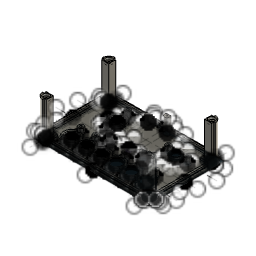
Cover_top v19 final (Autodesk Fusion 360 design; units mm, degrees)
Autodesk Fusion 360 part; units mm, degrees
(part 1 of 2)
sketch "Skizze1" plane through (0, 0, 0) normal (0, 0, 1) x (1, 0, 0)
  line L0 (85, -55) -> (-85, -55)
  line L1 (-85, -55) -> (-85, 55)
  line L2 (-85, 55) -> (85, 55)
  line L3 (85, 55) -> (85, -55)
  line L4 (85, -55) -> (-85, 55) construction
  line L5 (-85, -55) -> (85, 55) construction
  circle A0 centre (-75, 45) radius 10
  circle A1 centre (-75, -45) radius 10
  circle A2 centre (75, 45) radius 10
  line L6 (83.8, -53.8) -> (-83.8, -53.8)
  line L7 (-83.8, -53.8) -> (-83.8, 53.8)
  line L8 (-83.8, 53.8) -> (83.8, 53.8)
  line L9 (83.8, 53.8) -> (83.8, -53.8)
  line L10 (83.8, -53.8) -> (-83.8, 53.8) construction
  line L11 (-83.8, -53.8) -> (83.8, 53.8) construction
  line L12 (-70.8, 53.8) -> (-83.8, 53.8)
  line L13 (-83.8, 53.8) -> (-83.8, 40.8)
  line L14 (-83.8, 40.8) -> (-70.8, 40.8)
  line L15 (-70.8, 40.8) -> (-70.8, 53.8)
  line L16 (-83.8, 36) -> (-83.8, 45.2283)
  line L17 (-83.8, -40.8) -> (-70.8, -40.8)
  line L18 (-70.8, -40.8) -> (-70.8, -53.8)
  line L19 (-70.8, -53.8) -> (-83.8, -53.8)
  line L20 (-83.8, -53.8) -> (-83.8, -40.8)
  line L21 (83.8, -40.8) -> (70.8, -40.8)
  line L22 (70.8, -40.8) -> (70.8, -53.8)
  line L23 (70.8, -53.8) -> (83.8, -53.8)
  line L24 (83.8, -53.8) -> (83.8, -40.8)
  line L25 (70.8, 53.8) -> (83.8, 53.8)
  line L26 (83.8, 53.8) -> (83.8, 40.8)
  line L27 (83.8, 40.8) -> (70.8, 40.8)
  line L28 (70.8, 40.8) -> (70.8, 53.8)
  line L29 (-107.8935, 0) -> (101.4161, 0) construction
  line L30 (-81.6, -44) -> (-83.8, -44)
  line L31 (-83.8, -44) -> (-83.8, 44)
  line L32 (-83.8, 44) -> (-81.6, 44)
  line L33 (-81.6, 44) -> (-81.6, -44)
  line L34 (-81.6, -44) -> (-83.8, 44) construction
  line L35 (-83.8, -44) -> (-81.6, 44) construction
  line L36 (74, 51.6) -> (-74, 51.6)
  line L37 (-74, 51.6) -> (-74, 53.8)
  line L38 (-74, 53.8) -> (74, 53.8)
  line L39 (74, 53.8) -> (74, 51.6)
  line L40 (74, 51.6) -> (-74, 53.8) construction
  line L41 (-74, 51.6) -> (74, 53.8) construction
  line L42 (0, 66.6511) -> (0, -64.6622) construction
  line L43 (-89.5499, 46.3) -> (95, 46.3) construction
  line L44 (-93.2916, -46.3) -> (96.8462, -46.3) construction
  line L45 (-76.3, 67.4333) -> (-76.3, -70) construction
  line L46 (76.3, 67.4333) -> (76.3, -68.5532) construction
  circle A3 centre (76.3, -46.3) radius 4.5
  circle A4 centre (76.3, -46.3) radius 3
  circle A5 centre (76.3, 46.3) radius 4.5
  circle A6 centre (76.3, 46.3) radius 3
  circle A7 centre (-76.3, 46.3) radius 4.5
  circle A8 centre (-76.3, 46.3) radius 3
  circle A9 centre (-76.3, -46.3) radius 4.5
  circle A10 centre (-76.3, -46.3) radius 3
  line L47 (83.8, -44) -> (81.6, -44)
  line L48 (81.6, -44) -> (81.6, 44)
  line L49 (81.6, 44) -> (83.8, 44)
  line L50 (83.8, 44) -> (83.8, -44)
  line L51 (83.8, -44) -> (81.6, 44) construction
  line L52 (81.6, -44) -> (83.8, 44) construction
  line L53 (74, -53.8) -> (-74, -53.8)
  line L54 (-74, -53.8) -> (-74, -51.6)
  line L55 (-74, -51.6) -> (74, -51.6)
  line L56 (74, -51.6) -> (74, -53.8)
  line L57 (74, -53.8) -> (-74, -51.6) construction
  line L58 (-74, -53.8) -> (74, -51.6) construction
  line L59 (-95.9199, -30) -> (100, -30) construction
  line L60 (-91.3971, -16.03) -> (91.4123, -16.03) construction
  line L61 (-89.9566, -43.97) -> (89.6836, -43.97) construction
  line L62 (-11, 2.8713) -> (-11, -37.609) construction
  line L63 (-33, 11.0826) -> (-33, -38.4733) construction
  line L64 (-55, 10.5064) -> (-55, -36.1684) construction
  line L65 (11, 3.8797) -> (11, -36.4565) construction
  line L66 (33, 5.4644) -> (33, -35) construction
  line L67 (55, 5.8965) -> (55, -33.5753) construction
  circle A11 centre (-55, -30) radius 12
  circle A12 centre (-33, -30) radius 12
  circle A13 centre (-11, -30) radius 12
  circle A14 centre (11, -30) radius 12
  circle A15 centre (33, -30) radius 12
  circle A16 centre (55, -30) radius 12
  circle A17 centre (55, -16.03) radius 4
  circle A18 centre (33, -16.03) radius 4
  circle A19 centre (11, -16.03) radius 4
  circle A20 centre (-11, -16.03) radius 4
  circle A21 centre (-33, -16.03) radius 4
  circle A22 centre (-55, -16.03) radius 4
  circle A23 centre (-55, -43.97) radius 4
  circle A24 centre (-33, -43.97) radius 4
  circle A25 centre (-11, -43.97) radius 4
  circle A26 centre (11, -43.97) radius 4
  circle A27 centre (33, -43.97) radius 4
  circle A28 centre (55, -43.97) radius 4
  circle A29 centre (55, -30) radius 9.1
  circle A30 centre (55, -30) radius 8.1
  circle A31 centre (33, -30) radius 9.1
  circle A32 centre (33, -30) radius 8.1
  circle A33 centre (11, -30) radius 9.1
  circle A34 centre (11, -30) radius 8.1
  circle A35 centre (-11, -30) radius 9.1
  circle A36 centre (-11, -30) radius 8.1
  circle A37 centre (-33, -30) radius 9.1
  circle A38 centre (-33, -30) radius 8.1
  circle A39 centre (-55, -30) radius 9.1
  circle A40 centre (-55, -30) radius 8.1
  line L68 (-67.8, 37.8) -> (-67.8, 48.6)
  line L69 (-67.8, 48.6) -> (67.8, 48.6)
  line L70 (67.8, 48.6) -> (67.8, 37.8)
  line L71 (67.8, 37.8) -> (78.6, 37.8)
  line L72 (78.6, 37.8) -> (78.6, -37.8)
  line L73 (78.6, -37.8) -> (67.8, -37.8)
  line L74 (67.8, -37.8) -> (67.8, -48.6)
  line L75 (67.8, -48.6) -> (-67.8, -48.6)
  line L76 (-67.8, -48.6) -> (-67.8, -38.0603)
  line L77 (-67.8, -38.0603) -> (-78.6, -38.0603)
  line L78 (-78.6, -38.0603) -> (-78.6, 37.8)
  line L79 (-78.6, 37.8) -> (-67.8, 37.8)
  line L80 (-100.7551, 25) -> (105, 25) construction
  line L81 (44.54, 42.8921) -> (44.54, 3.8544) construction
  line L82 (-42, 44.1013) -> (-42, 5.0635) construction
  circle A41 centre (-42, 25) radius 9.1
  circle A42 centre (-42, 25) radius 8.1
  circle A43 centre (-42, 25) radius 12
  line L83 (-48.7348, 40.24) -> (-29.0042, 40.24) construction
  line L84 (-50, 9.76) -> (-24.2465, 9.76) construction
  circle A44 centre (-42, 40.24) radius 4
  circle A45 centre (-42, 9.76) radius 4
  circle A46 centre (44.54, 25) radius 6.25
  circle A47 centre (44.54, 25) radius 7.5
  line L85 (61.54, 32) -> (61.54, 15) construction
  line L86 (33.54, 36) -> (33.54, 15.2872) construction
  circle A48 centre (33.54, 25) radius 4
  circle A49 centre (61.54, 25) radius 4
  line L87 (-55.79, 35.0443) -> (-55.79, 15.0443) construction
  circle A50 centre (-55.79, 25) radius 3.25
  circle A51 centre (-55.79, 25) radius 1.75
  line L88 (-22.9425, -17) -> (36.8868, -17) construction
  line L89 (-26.9921, 49.1) -> (29.3101, 49.1) construction
  line L90 (-28, 65.5218) -> (-28, -4.3972) construction
  line L91 (-25.5, 61.3213) -> (-25.5, -3.5842) construction
  line L92 (-20.4, 60) -> (-20.4, -2) construction
  line L93 (7.5, 61) -> (7.5, 1) construction
  line L94 (22.7, 60.5796) -> (22.7, -4.8964) construction
  line L95 (3.5, 51.6) -> (11.5, 51.6)
  line L96 (11.5, 51.6) -> (11.5, 45.1) construction
  line L97 (11.5, 45.1) -> (3.5, 45.1) construction
  line L98 (3.5, 45.1) -> (3.5, 51.6) construction
  line L99 (-24.4, 51.6) -> (-16.4, 51.6)
  line L100 (-16.4, 51.6) -> (-16.4, 45.1) construction
  line L101 (-16.4, 45.1) -> (-24.4, 45.1) construction
  line L102 (-24.4, 45.1) -> (-24.4, 51.6) construction
  line L103 (-17.4, 51.6) -> (-17.4, 45.1)
  arc A52 (-24.4, 49.1) -> (-16.4, 49.1) centre (-20.4, 49.1) ccw
  arc A53 (-23.5225, 51.6) -> (-24.4, 49.1) centre (-20.4, 49.1) ccw
  arc A54 (-16.4, 49.1) -> (-17.2775, 51.6) centre (-20.4, 49.1) ccw
  arc A55 (3.5, 49.1) -> (10.6225, 51.6) centre (7.5, 49.1) ccw
  arc A56 (4.3775, 51.6) -> (3.5, 49.1) centre (7.5, 49.1) ccw
  line L104 (18, -1.7) -> (26.495, -1.7) construction
  line L105 (27, -3) -> (-31, -3) construction
  circle A57 centre (22.7, -1.7) radius 4
  circle A58 centre (-25.5, -3) radius 4
  line L106 (19.3593, 0.5) -> (26.0407, 0.5)
  line L107 (74.2, -53.6) -> (74.2, -51.4)
  line L108 (74.2, -51.4) -> (71, -51.4)
  line L109 (71, -51.4) -> (71, -41)
  line L110 (71, -41) -> (81.4, -41)
  line L111 (81.4, -41) -> (81.4, -44.2)
  line L112 (81.4, -44.2) -> (83.6, -44.2)
  line L113 (74, -54.6568) -> (74, -41.9102) construction
  line L114 (69.7927, -44) -> (87.5, -44) construction
  arc A59 (74, -53.8) -> (83.8, -44) centre (74, -44) ccw
  arc A60 (74.2, -53.6) -> (83.6, -44.2) centre (74, -44) ccw
  line L115 (72.8, -53.6) -> (76.6, -53.6) construction
  line L116 (83.6, -43.5) -> (83.6, -45.7322) construction
  circle A61 centre (75, -45) radius 10
  arc A62 (-83.6, -44.2) -> (-74.2, -53.6) centre (-74, -44) ccw
  line L117 (-74.2, -53.6) -> (-74.2, -51.4)
  line L118 (-74.2, -51.4) -> (-71, -51.4)
  line L119 (-71, -41) -> (-81.4, -41)
  line L120 (-81.4, -41) -> (-81.4, -44.2)
  line L121 (-81.4, -44.2) -> (-83.6, -44.2)
  line L122 (-71, -51.4) -> (-71, -41)
  arc A63 (-83.8, -44) -> (-74, -53.8) centre (-74, -44) ccw
  arc A64 (-74.2, 53.6) -> (-83.6, 44.2) centre (-74, 44) ccw
  line L123 (-74.2, 53.6) -> (-74.2, 51.4)
  line L124 (-74.2, 51.4) -> (-71, 51.4)
  line L125 (-71, 41) -> (-81.4, 41)
  line L126 (-81.4, 41) -> (-81.4, 44.2)
  line L127 (-81.4, 44.2) -> (-83.6, 44.2)
  line L128 (-71, 51.4) -> (-71, 41)
  arc A65 (-74, 53.8) -> (-83.8, 44) centre (-74, 44) ccw
  arc A66 (83.6, 44.2) -> (74.2, 53.6) centre (74, 44) ccw
  line L129 (74.2, 53.6) -> (74.2, 51.4)
  line L130 (74.2, 51.4) -> (71, 51.4)
  line L131 (71, 41) -> (81.4, 41)
  line L132 (81.4, 41) -> (81.4, 44.2)
  line L133 (81.4, 44.2) -> (83.6, 44.2)
  line L134 (71, 51.4) -> (71, 41)
  arc A67 (83.8, 44) -> (74, 53.8) centre (74, 44) ccw
  line L135 (-83.6, 44.2) -> (-83.8, 44.2)
  line L136 (-74.2, 53.6) -> (-74.2, 53.8)
  line L137 (74.2, 53.6) -> (74.2, 53.8)
  line L138 (83.6, 44.2) -> (83.8, 44.2)
  line L139 (83.6, -44.2) -> (83.8, -44.2)
  line L140 (74.2, -53.6) -> (74.2, -53.8)
  line L141 (-74.2, -53.6) -> (-74.2, -53.8)
  line L142 (-83.6, -44.2) -> (-83.8, -44.2)
  line L143 (-11.75, 70) -> (-11.75, 19) construction
  point P0 (-82.7, 0)
  point P1 (0, 52.7)
  point P2 (76.3, -46.3)
  point P3 (76.3, 46.3)
  point P4 (-76.3, 46.3)
  point P5 (-76.3, -46.3)
  point P6 (82.7, 0)
  point P7 (0, -52.7)
  point P8 (-55, -30)
  point P9 (-33, -30)
  point P10 (-11, -30)
  point P11 (11, -30)
  point P12 (33, -30)
  point P13 (55, -30)
  point P14 (-55, -16.03)
  point P15 (-33, -16.03)
  point P16 (-11, -16.03)
  point P17 (11, -16.03)
  point P18 (33, -16.03)
  point P19 (55, -16.03)
  point P20 (55, -43.97)
  point P21 (33, -43.97)
  point P22 (11, -43.97)
  point P23 (-11, -43.97)
  point P24 (-33, -43.97)
  point P25 (-55, -43.97)
  point P26 (-42, 25)
  point P27 (44.54, 25)
  point P28 (-42, 9.76)
  point P29 (-42, 40.24)
  point P30 (33.54, 25)
  point P31 (61.54, 25)
  point P32 (7.5, 49.1)
  point P33 (-20.4, 49.1)
  point P34 (-25.5, -3)
  point P35 (22.7, -1.7)
  point P36 (74.2, -44.2)
  point P37 (74, -44)
  point P38 (74.2, -53.6)
  point P39 (83.6, -44.2)
  dimension "d1" = 110
  dimension "d2" = 170
  dimension "d3" = 20
  dimension "d4" = 20
  dimension "d6" = 20
  dimension "d7" = 167.6
  dimension "d8" = 107.6
  dimension "d13" = 13
  dimension "d14" = 13
  dimension "d17" = 13
  dimension "d18" = 13
  dimension "d19" = 13
  dimension "d20" = 13
  dimension "d21" = 13
  dimension "d22" = 13
  dimension "d23" = 1.1
  dimension "d24" = 2.2
  dimension "d25" = 88
  dimension "d26" = 1.1
  dimension "d27" = 2.2
  dimension "d28" = 148
  dimension "d29" = 5.5
  dimension "d30" = 5.5
  dimension "d31" = 5.5
  dimension "d32" = 5.5
  dimension "d33" = 9
  dimension "d34" = 6
  dimension "d35" = 9
  dimension "d36" = 6
  dimension "d37" = 6
  dimension "d38" = 9
  dimension "d39" = 6
  dimension "d40" = 9
  dimension "d41" = 2.2
  dimension "d42" = 1.1
  dimension "d43" = 88
  dimension "d44" = 1.1
  dimension "d45" = 148
  dimension "d46" = 2.2
  dimension "d47" = 25
  dimension "d48" = 13.97
  dimension "d49" = 13.97
  dimension "d50" = 11
  dimension "d51" = 22
  dimension "d52" = 22
  dimension "d53" = 11
  dimension "d54" = 22
  dimension "d55" = 22
  dimension "d56" = 24
  dimension "d57" = 24
  dimension "d58" = 24
  dimension "d59" = 24
  dimension "d60" = 24
  dimension "d61" = 24
  dimension "d62" = 8
  dimension "d63" = 8
  dimension "d64" = 8
  dimension "d65" = 8
  dimension "d66" = 8
  dimension "d67" = 8
  dimension "d68" = 8
  dimension "d69" = 8
  dimension "d70" = 8
  dimension "d71" = 8
  dimension "d72" = 8
  dimension "d73" = 8
  dimension "d74" = 18.2
  dimension "d75" = 18.2
  dimension "d76" = 18.2
  dimension "d77" = 18.2
  dimension "d78" = 18.2
  dimension "d79" = 18.2
  dimension "d80" = 16.2
  dimension "d81" = 16.2
  dimension "d82" = 16.2
  dimension "d83" = 16.2
  dimension "d84" = 16.2
  dimension "d85" = 16.2
  dimension "d116" = 3
  dimension "d117" = 3
  dimension "d118" = 3
  dimension "d119" = 3
  dimension "d120" = 3
  dimension "d121" = 3
  dimension "d122" = 3
  dimension "d123" = 3
  dimension "d124" = 3
  dimension "d125" = 3
  dimension "d126" = 3
  dimension "d127" = 2.7397
  dimension "d130" = 30
  dimension "d131" = 42
  dimension "d132" = 44.54
  dimension "d133" = 18.2
  dimension "d134" = 16.2
  dimension "d135" = 24
  dimension "d136" = 15.24
  dimension "d137" = 15.24
  dimension "d138" = 8
  dimension "d139" = 8
  dimension "d140" = 12.5
  dimension "d141" = 15
  dimension "d142" = 17
  dimension "d143" = 11
  dimension "d144" = 8
  dimension "d145" = 8
  dimension "d214" = 6.5
  dimension "d215" = 3.5
  dimension "d220" = 135.6
  dimension "d221" = 5.5
  dimension "d222" = 5.5
  dimension "d223" = 7.5
  dimension "d224" = 3.2
  dimension "d225" = 13.79
  dimension "d227" = 66.1
  dimension "d228" = 68.6
  dimension "d229" = 2.5
  dimension "d230" = 28
  dimension "d231" = 2.5
  dimension "d232" = 5.1
  dimension "d233" = 27.9
  dimension "d234" = 15.2
  dimension "d235" = 48.2
  dimension "d236" = 4
  dimension "d237" = 4
  dimension "d238" = 4
  dimension "d240" = 4
  dimension "d241" = 4
  dimension "d242" = 4
  dimension "d243" = 3
  dimension "d244" = 50.8
  dimension "d245" = 1.3
  dimension "d246" = 8
  dimension "d247" = 8
  dimension "d248" = 2.2
  dimension "d256" = 49.1
  dimension "d279" = 76.3
  dimension "d282" = 46.3
  dimension "d306" = 0.2
  dimension "d307" = 0.2
  dimension "d308" = 0.2
  dimension "d309" = 0.2
  dimension "d312" = 0.2
  dimension "d313" = 0.2
  dimension "d314" = 0.2
  dimension "d315" = 0.2
  dimension "d316" = 20
  dimension "d333" = 3.2
  dimension "d334" = 14.2
  dimension "d335" = 14.2
  dimension "d336" = 92.6
  dimension "d337" = 11.36
  dimension "d338" = 16.25
  dimension "d339" = 62.25
  dimension "d340" = 32
  constraint horizontal L0
  constraint perpendicular L0 L1
  constraint parallel L0 L2
  constraint parallel L1 L3
  constraint coincident L4 origin
  constraint coincident L5 origin
  constraint tangent L2 A0
  constraint tangent L1 A0
  constraint tangent L1 A1
  constraint tangent L0 A1
  constraint tangent L2 A2
  constraint tangent L3 A2
  constraint horizontal L6
  constraint perpendicular L6 L7
  constraint parallel L6 L8
  constraint parallel L7 L9
  constraint coincident L10 origin
  constraint coincident L11 origin
  constraint horizontal L12
  constraint vertical L13
  constraint horizontal L14
  constraint vertical L15
  constraint coincident L7 L13.end
  constraint coincident L8 L12.start
  constraint vertical L16
  constraint coincident L7 L16.end
  constraint horizontal L17
  constraint vertical L18
  constraint horizontal L19
  constraint vertical L20
  constraint coincident L6 L18.end
  constraint coincident L7 L17.start
  constraint horizontal L21
  constraint vertical L22
  constraint horizontal L23
  constraint vertical L24
  constraint coincident L6 L22.end
  constraint coincident L9 L21.start
  constraint horizontal L25
  constraint vertical L26
  constraint horizontal L27
  constraint vertical L28
  constraint coincident L9 L26.end
  constraint coincident L8 L25.start
  constraint perpendicular L3 L29
  constraint coincident origin L29
  constraint horizontal L30
  constraint perpendicular L30 L31
  constraint parallel L30 L32
  constraint parallel L31 L33
  constraint coincident L34 P0
  constraint coincident L35 P0
  constraint coincident L29 P0
  constraint horizontal L36
  constraint perpendicular L36 L37
  constraint parallel L36 L38
  constraint parallel L37 L39
  constraint coincident L40 P1
  constraint coincident L41 P1
  constraint perpendicular L0 L42
  constraint coincident origin L42
  constraint coincident P1 L42
  constraint parallel L36 L43
  constraint perpendicular L1 L44
  constraint perpendicular L17 L45
  constraint perpendicular L0 L46
  constraint coincident L44 P2
  constraint coincident L46 P2
  constraint coincident P2 A3.centre
  constraint coincident L43 P3
  constraint coincident L46 P3
  constraint coincident P3 A5.centre
  constraint coincident L43 P4
  constraint coincident L45 P4
  constraint coincident P4 A7.centre
  constraint coincident L44 P5
  constraint coincident L45 P5
  constraint coincident P5 A9.centre
  constraint horizontal L47
  constraint perpendicular L47 L48
  constraint parallel L47 L49
  constraint parallel L48 L50
  constraint coincident L51 P6
  constraint coincident L52 P6
  constraint coincident L29 P6
  constraint horizontal L53
  constraint perpendicular L53 L54
  constraint parallel L53 L55
  constraint parallel L54 L56
  constraint coincident L57 P7
  constraint coincident L58 P7
  constraint coincident L42 P7
  constraint perpendicular L3 L59
  constraint perpendicular L3 L60
  constraint perpendicular L50 L61
  constraint perpendicular L44 L62
  constraint perpendicular L61 L63
  constraint perpendicular L61 L64
  constraint perpendicular L61 L65
  constraint perpendicular L60 L66
  constraint vertical L67
  constraint coincident L59 P8
  constraint coincident L64 P8
  constraint coincident L59 P9
  constraint coincident L63 P9
  constraint coincident L59 P10
  constraint coincident L62 P10
  constraint coincident L59 P11
  constraint coincident L65 P11
  constraint coincident L59 P12
  constraint coincident L66 P12
  constraint coincident L59 P13
  constraint coincident L67 P13
  constraint coincident L60 P14
  constraint coincident L64 P14
  constraint coincident L60 P15
  constraint coincident L63 P15
  constraint coincident L60 P16
  constraint coincident L62 P16
  constraint coincident L60 P17
  constraint coincident L65 P17
  constraint coincident L66 P18
  constraint coincident L60 P18
  constraint coincident L60 P19
  constraint coincident L67 P19
  constraint coincident L61 P20
  constraint coincident L67 P20
  constraint coincident L66 P21
  constraint coincident L61 P21
  constraint coincident L61 P22
  constraint coincident L65 P22
  constraint coincident L61 P23
  constraint coincident L62 P23
  constraint coincident L61 P24
  constraint coincident L63 P24
  constraint coincident L61 P25
  constraint coincident L64 P25
  constraint coincident P8 A11.centre
  constraint coincident P9 A12.centre
  constraint coincident P10 A13.centre
  constraint coincident P11 A14.centre
  constraint coincident P12 A15.centre
  constraint coincident P13 A16.centre
  constraint coincident P19 A17.centre
  constraint coincident P18 A18.centre
  constraint coincident P17 A19.centre
  constraint coincident P16 A20.centre
  constraint coincident P15 A21.centre
  constraint coincident P14 A22.centre
  constraint coincident P25 A23.centre
  constraint coincident P24 A24.centre
  constraint coincident P23 A25.centre
  constraint coincident P22 A26.centre
  constraint coincident P21 A27.centre
  constraint coincident P20 A28.centre
  constraint concentric A16 A29
  constraint concentric A15 A31
  constraint concentric A15 A32
  constraint concentric A14 A34
  constraint perpendicular L43 L68
  constraint perpendicular L28 L69
  constraint perpendicular L43 L70
  constraint perpendicular L46 L71
  constraint perpendicular L71 L72
  constraint perpendicular L46 L73
  constraint perpendicular L44 L74
  constraint perpendicular L74 L75
  constraint coincident A1 L76.end
  constraint perpendicular L75 L76
  constraint perpendicular L45 L77
  constraint perpendicular L77 L78
  constraint perpendicular L68 L79
  constraint perpendicular L3 L80
  constraint perpendicular L43 L81
  constraint coincident L80 P26
  constraint coincident L82 P26
  constraint coincident L80 P27
  constraint coincident L81 P27
  constraint coincident P26 A41.centre
  constraint perpendicular L45 L83
  constraint horizontal L84
  constraint coincident L82 P28
  constraint coincident L84 P28
  constraint coincident L82 P29
  constraint coincident L83 P29
  constraint coincident P29 A44.centre
  constraint coincident P28 A45.centre
  constraint coincident P27 A46.centre
  constraint perpendicular L80 L85
  constraint perpendicular L80 L86
  constraint coincident L80 P30
  constraint coincident L86 P30
  constraint coincident L80 P31
  constraint coincident L85 P31
  constraint coincident P30 A48.centre
  constraint coincident P31 A49.centre
  constraint perpendicular L80 L87
  constraint coincident L80 A50.centre
  constraint coincident L87 A50.centre
  constraint concentric A50 A51
  constraint perpendicular L66 L88
  constraint parallel L43 L89
  constraint perpendicular L2 L90
  constraint perpendicular L29 L91
  constraint perpendicular L29 L92
  constraint vertical L93
  constraint perpendicular L29 L94
  constraint horizontal L95
  constraint vertical L96
  constraint horizontal L97
  constraint vertical L98
  constraint coincident L36 L95.start
  constraint coincident L89 P32
  constraint coincident L93 P32
  constraint coincident L92 P33
  constraint coincident L89 P33
  constraint horizontal L99
  constraint vertical L100
  constraint horizontal L101
  constraint vertical L102
  constraint coincident L36 L99.start
  constraint coincident L36 L103.start
  constraint coincident L101 L103.end
  constraint perpendicular L101 L103
  constraint coincident L100 A52.end
  constraint coincident L89 A52.start
  constraint coincident L102 A52.start
  constraint coincident P33 A52.centre
  constraint coincident L99 A53.start
  constraint coincident L99 A54.end
  constraint coincident L95 A55.end
  constraint coincident L89 A55.start
  constraint coincident L98 A55.start
  constraint coincident P32 A55.centre
  constraint coincident L95 A56.start
  constraint perpendicular L94 L104
  constraint perpendicular L90 L105
  constraint coincident L105 P34
  constraint coincident L91 P34
  constraint coincident L104 P35
  constraint coincident L94 P35
  constraint coincident P35 A57.centre
  constraint coincident P34 A58.centre
  constraint coincident A57 L106.start
  constraint coincident A57 L106.end
  constraint parallel L29 L106
  constraint perpendicular L23 L107
  constraint perpendicular L107 L108
  constraint perpendicular L109 L110
  constraint perpendicular L61 L111
  constraint perpendicular L111 L112
  constraint perpendicular L61 L113
  constraint coincident L55.end L113
  constraint perpendicular L3 L114
  constraint coincident L47.end L114
  constraint coincident L113 P37
  constraint coincident L114 P37
  constraint coincident P37 A59.centre
  constraint perpendicular L46 L115
  constraint coincident P38 L107.start
  constraint perpendicular L61 L116
  constraint coincident P39 L112.end
  constraint tangent L0 A61
  constraint tangent L3 A61
  constraint symmetric L42 L53.start L53.end
  constraint symmetric L42 L109.end L119.start
  constraint symmetric L42 P38 A62.end
  constraint symmetric L42 L107.end L117.end
  constraint symmetric L42 L108.end L118.end
  constraint symmetric L42 L110.end L119.end
  constraint symmetric L42 L111.end L120.end
  constraint symmetric L42 P39 A62.start
  constraint symmetric L42 L47.start L30.end
  constraint symmetric L42 A59 A63
  constraint symmetric L42 A60 A62
  constraint symmetric L29 L53.start L38.end
  constraint symmetric L29 L109.end L131.start
  constraint symmetric L29 P38 A66.end
  constraint symmetric L29 L107.end L129.end
  constraint symmetric L29 L108.end L130.end
  constraint symmetric L29 L110.end L131.end
  constraint symmetric L29 L111.end L132.end
  constraint symmetric L29 P39 A66.start
  constraint symmetric L29 L47.start L49.end
  constraint symmetric L29 A59 A67
  constraint symmetric L29 A60 A66
  constraint symmetric L29 A62.end A64.start
  constraint symmetric L29 A62.start A64.end
  constraint symmetric L29 A62 A64
  constraint symmetric L29 L117.end L123.end
  constraint symmetric L29 L118.end L124.end
  constraint symmetric L29 L119.start L125.start
  constraint symmetric L29 L119.end L125.end
  constraint symmetric L29 L120.end L126.end
  constraint symmetric L29 L53.end L37.end
  constraint symmetric L29 L30.end L31.end
  constraint symmetric L29 A63 A65
  constraint coincident L7 L135.end
  constraint coincident L12 L136.end
  constraint coincident L25 L137.end
  constraint coincident L9 L138.end
  constraint coincident L9 L139.end
  constraint coincident L23 L140.end
  constraint coincident L6 L141.end
  constraint coincident L7 L142.end
  constraint perpendicular L80 L143
  measures "d1" distance of L0 L2
  measures "d2" distance of L1 L3
  measures "d3" diameter of A0
  measures "d4" diameter of A2
  measures "d6" diameter of A1
  measures "d7" distance of L7 L9
  measures "d8" distance of L6 L8
  measures "d13" distance of L7 L15
  measures "d14" distance of L8 L14
  measures "d17" distance of L9 L28
  measures "d18" distance of L8 L27
  measures "d19" distance of L6 L21
  measures "d20" distance of L9 L22
  measures "d21" distance of L6 L17
  measures "d22" distance of L7 L18
  measures "d23" distance of L7 P0
  measures "d24" distance of L31 L33
  measures "d25" distance of L30 L32
  measures "d26" distance of L8 P1
  measures "d27" distance of L36 L38
  measures "d28" distance of L37 L39
  measures "d29" distance of L27 L43
  measures "d30" distance of L21 L44
  measures "d31" distance of L18 L45
  measures "d32" distance of L22 L46
  measures "d33" diameter of A3
  measures "d34" diameter of A4
  measures "d35" diameter of A5
  measures "d36" diameter of A6
  measures "d37" diameter of A8
  measures "d38" diameter of A7
  measures "d39" diameter of A10
  measures "d40" diameter of A9
  measures "d41" distance of L48 L50
  measures "d42" distance of L9 P6
  measures "d43" distance of L47 L49
  measures "d44" distance of L6 P7
  measures "d45" distance of L54 L56
  measures "d46" distance of L53 L55
  measures "d47" distance of L0 L59
  measures "d48" distance of L59 L60
  measures "d49" distance of L59 L61
  measures "d50" distance of L42 L62
  measures "d51" distance of L62 L63
  measures "d52" distance of L63 L64
  measures "d53" distance of L42 L65
  measures "d54" distance of L65 L66
  measures "d55" distance of L66 L67
  measures "d56" diameter of A11
  measures "d57" diameter of A12
  measures "d58" diameter of A13
  measures "d59" diameter of A14
  measures "d60" diameter of A15
  measures "d61" diameter of A16
  measures "d62" diameter of A22
  measures "d63" diameter of A21
  measures "d64" diameter of A20
  measures "d65" diameter of A19
  measures "d66" diameter of A18
  measures "d67" diameter of A17
  measures "d68" diameter of A28
  measures "d69" diameter of A27
  measures "d70" diameter of A26
  measures "d71" diameter of A25
  measures "d72" diameter of A24
  measures "d73" diameter of A23
  measures "d74" diameter of A29
  measures "d75" diameter of A31
  measures "d76" diameter of A33
  measures "d77" diameter of A35
  measures "d78" diameter of A37
  measures "d79" diameter of A39
  measures "d80" diameter of A40
  measures "d81" diameter of A38
  measures "d82" diameter of A36
  measures "d83" diameter of A34
  measures "d84" diameter of A32
  measures "d85" diameter of A30
  measures "d116" distance of L14 L79
  measures "d117" distance of L33 L78
  measures "d118" distance of L15 L68
  measures "d119" distance of L36 L69
  measures "d120" distance of L28 L70
  measures "d121" distance of L27 L71
  measures "d122" distance of L48 L72
  measures "d123" distance of L21 L73
  measures "d124" distance of L22 L74
  measures "d125" distance of L55 L75
  measures "d126" distance of L18 L76
  measures "d127" distance of L17 L77
  measures "d130" distance of L2 L80
  measures "d131" distance of L42 L82
  measures "d132" distance of L42 L81
  measures "d133" diameter of A41
  measures "d134" diameter of A42
  measures "d135" diameter of A43
  measures "d136" distance of L80 L83
  measures "d137" distance of L80 L84
  measures "d138" diameter of A44
  measures "d139" diameter of A45
  measures "d140" diameter of A46
  measures "d141" diameter of A47
  measures "d142" distance of L81 L85
  measures "d143" distance of L81 L86
  measures "d144" diameter of A49
  measures "d145" diameter of A48
  measures "d214" diameter of A50
  measures "d215" diameter of A51
  measures "d220" distance of L74 L76
  measures "d221" distance of L15 P4
  measures "d222" distance of L14 P4
  measures "d223" distance of L13 P4
  measures "d224" distance of L15 L37
  measures "d225" distance of L82 L87
  measures "d227" distance of L88 L89
  measures "d228" distance of L36 L88
  measures "d229" distance of L36 L89.end
  measures "d230" distance of L42 L90
  measures "d231" distance of L90 L91
  measures "d232" distance of L91 L92
  measures "d233" distance of L92 L93
  measures "d234" distance of L93 L94
  measures "d235" distance of L91 L94
  measures "d236" distance of L93 L98
  measures "d237" distance of L93 L96
  measures "d238" distance of L89 L97
  measures "d240" distance of P33 L100
  measures "d241" distance of P33 L102
  measures "d242" distance of L89 L101
  measures "d243" distance of L92 L103
  measures "d244" distance of L89 L104
  measures "d245" distance of L104 L105
  measures "d246" diameter of A58
  measures "d247" diameter of A57
  measures "d248" distance of L104 L106
  measures "d256" vertical distance of origin P32
  measures "d279" distance of origin L46
  measures "d282" distance of origin L43
  measures "d306" distance of L21 L110
  measures "d307" distance of L22 L109
  measures "d308" distance of L55 L108
  measures "d309" distance of L56 L107
  measures "d312" distance of L47 L112
  measures "d313" distance of L48 L111
  measures "d314" distance of L23 L115
  measures "d315" distance of L24 L116
  measures "d316" diameter of A61
  measures "d333" distance of L22 L55.end
  measures "d334" distance of L0.start L22
  measures "d335" distance of L0.start L21
  measures "d336" distance of P2 P3
  measures "d337" distance of L36 P29
  measures "d338" distance of L90 L143
  measures "d339" distance of L37 L143
  measures "d340" distance of L37 P29
extrude "Extrusion1" add sketch "Skizze1" along normal blind 5 contours L0 A1 L6 L53 A61 | L6 L23 L53 A61 | L3 A2 L9 L50 A61 | L9 L24 L50 A61 | A1 L6 L19 L53 | L6 L9 L23 L24 A59 A61 L139 L140 | A2 L9 L26 L50 | A1 L6 L7 L19 L20 A63 L141 L142 | L6 L23 A59 L140 | A2 L8 L9 L25 L26 A67 L137 L138 | L9 L24 A59 L139 | L1 A0 A1 L7 L16 L31 | A1 L7 L20 L31 | L6 L19 A63 L141 | A59 A60 L139 L140 | L2 A0 A2 L8 L38 | A2 L8 L25 L38 | L9 L26 A67 L138 | A0 L7 L13 L16 L31 | L7 L20 A63 L142 | A62 A63 L141 L142 | A0 L8 L12 L38 | L8 L25 A67 L137 | A66 A67 L137 L138 | A0 L7 L8 L12 L13 L16 A65 L135 L136 | L8 L12 A65 L136 | L7 L13 L16 A65 L135 | A64 A65 L135 L136 makes body 1
extrude "Extrusion2" add sketch "Skizze1" along normal blind 2 contours L6 L22 L53 L55 A61 | A1 L6 L53 L55 A61 | L6 L9 L23 L24 A59 A61 | A2 L9 L48 L50 A61 | L9 L21 L48 L50 A61 | A1 L6 L7 L19 L20 A63 | A1 L6 L18 L53 L55 | L6 L22 L23 L53 L55 L56 | A59 A60 L139 L140 | L6 L9 L21 L22 L23 L24 L47 L48 L55 L56 L107 L108 L109 L110 L111 L112 A59 L139 L140 | A2 L8 L9 L25 L26 A67 | A2 L9 L27 L48 L50 | L9 L21 L24 L47 L48 L50 | L6 L7 L17 L18 L19 L20 L30 L33 L54 L55 L117 L118 L119 L120 L121 L122 A63 L141 L142 | A62 A63 L141 L142 | L6 L18 L19 L53 L54 L55 | L74 L75 A61 | A0 A1 A2 L68 L69 L70 L71 L72 L73 L74 L75 L78 L79 A52 A55 A61 | L107 L108 L109 L110 L111 L112 A60 | A66 A67 L137 L138 | L8 L9 L25 L26 L27 L28 L36 L39 L48 L49 L129 L130 L131 L132 L133 L134 A67 L137 L138 | L9 L26 L27 L48 L49 L50 | L72 L73 A61 | A0 A1 L7 L16 L31 L33 | A1 L7 L17 L31 L33 | A62 L117 L118 L119 L120 L121 L122 | A1 L75 L76 | A2 L8 L28 L36 L38 | A0 A2 L8 L36 L38 L95 L99 | A66 L129 L130 L131 L132 L133 L134 | A2 L71 L72 | A0 L7 L8 L12 L13 L16 A65 | A0 L7 L14 L16 L31 L33 | L7 L17 L20 L30 L31 L33 | A0 L8 L15 L36 L38 | L8 L25 L28 L36 L38 L39 | L7 L13 L14 L16 L31 L32 L33 | A1 L77 L78 | L8 L12 L15 L36 L37 L38 | A64 A65 L135 L136 | L7 L8 L12 L13 L14 L15 L16 L32 L33 L36 L37 L123 L124 L125 L126 L127 L128 A65 L135 L136 | A2 L69 L70 | A0 L78 L79 | A0 L68 L69 | A64 L123 L124 L125 L126 L127 L128 | L69 A55 | L69 L103 A52 | L69 L103 A52 | A3 | A4 | A5 | A6 | A7 | A8 | A9 | A10 | A29 | A31 | A33 | A35 | A37 | A39 | A41 | A57 L106 | A57 L106 | A58 bodies 1 makes body 2 at (-1.9113, -30.4536, 1.3333) makes body 3 at (20.0887, -30.4536, 1.3333) makes body 4 at (-23.9113, -30.4536, 1.3333) makes body 5 at (64.0887, -30.4536, 1.3333) makes body 6 at (42.0887, -30.4536, 1.3333) makes body 7 at (-45.9113, -30.4536, 1.3333) makes body 8 at (-32.9113, 24.5464, 1.3333) makes body 9 at (-3.4962, 11.4306, 0)
extrude "Extrusion8" add sketch "Skizze1" along normal blind 5 contours L21 L22 L48 L55 L72 L73 L74 L75 A61 | A1 L55 L75 A61 | A2 L48 L72 A61 | A1 L17 L18 L33 L55 L75 L76 L77 L78 | A2 L27 L28 L36 L48 L69 L70 L71 L72 | L73 L74 A61 | A0 A1 L33 L78 | A2 L36 L69 L95 A55 | A2 L70 L71 | A0 L14 L15 L33 L36 L68 L69 L78 L79 | A0 L36 L69 L99 A52 A53 | L36 L69 L95 A55 A56 | A0 L68 L79 | L36 L69 L99 L103 A52 A53 | L36 L69 L95 L99 A52 A54 A55 A56 | L36 L69 L99 L103 A52 A54 bodies 9 1
extrude "Extrusion4" add sketch "Skizze1" along normal blind 5 separate body contours A11 A12 | A11 A12 A13 A21 A24 | A11 A12 A22 A23 | A12 A13 A14 A20 A25 | A12 A13 | A13 A14 A15 A19 A26 | A13 A14 | A14 A15 A16 A18 A27 | A14 A15 | A15 A16 A17 A28 | A15 A16 | A43 A44 A45 A50 | A47 A48 picked at (37.7663, 22.9753) makes body 10 at (44, -27.4972, 0) makes body 11 at (-32.9113, 24.5464, 3.3333) makes body 12 at (37.4003, 22.7034, 3.3333)
extrude "Extrusion5" add sketch "Skizze1" along normal blind 10.3 separate body contours A11 A22 | A11 A22 | A12 A21 | A12 A21 | A11 A23 | A11 A23 | A12 A24 | A12 A24 | A13 A20 | A13 A20 | A13 A25 | A13 A25 | A14 A19 | A14 A19 | A14 A26 | A14 A26 | A15 A18 | A15 A18 | A15 A27 | A15 A27 | A16 A17 | A16 A17 | A16 A28 | A16 A28 | A47 A48 | A47 A48 | A49 picked at (37.2193, 25) picked at (34.5563, 25.0984) makes body 13 at (-51.0199, -44.3683, 3.4333) makes body 14 at (-7.0199, -44.3683, 3.4333) makes body 15 at (36.9801, -44.3683, 3.4333) makes body 16 at (58.9801, -44.3683, 3.4333) makes body 17 at (14.9801, -43.5717, 6.8667) makes body 18 at (-29.0199, -43.5717, 6.8667) makes body 19 at (37.5201, 24.6017, 3.4333) makes body 20 at (-51.0199, -15.6317, 6.8667) makes body 21 at (-7.0199, -15.6317, 6.8667) makes body 22 at (36.9801, -15.6317, 6.8667) makes body 23 at (58.9801, -15.6317, 6.8667) makes body 24 at (14.9801, -15.6317, 6.8667) makes body 25 at (-29.0199, -15.6317, 6.8667) makes body 26 at (65.535, 24.8006, 6.8667)
extrude "Extrusion10" add sketch "Skizze1" along normal blind 10.3 contours A43 A44 | A43 A44 | A43 A45 | A43 A45 bodies 11 9
sketch "Skizze3" plane through (0, 0, 10.3) normal (0, 0, 1) x (-1, 0, 0)
  circle A0 centre (-33.54, -25) radius 4
  line L0 (-14, -25) -> (-75.6564, -25) construction
  line L1 (85, -55) -> (-85, -55)
  line L2 (-33.54, -35) -> (-33.54, -8) construction
  line L3 (-44.54, -42.8921) -> (-44.54, -3.8544)
  line L4 (-61.54, -38) -> (-61.54, -6) construction
  line L5 (72, 30) -> (-73, 30) construction
  line L6 (68, 16.03) -> (-75, 16.03) construction
  line L7 (97, 43.97) -> (-63, 43.97) construction
  line L8 (11, 9) -> (11, 49) construction
  line L9 (33, 9) -> (33, 52) construction
  line L10 (55, 8) -> (55, 52) construction
  line L11 (-11, 9) -> (-11, 49.4628) construction
  line L12 (-33, 8) -> (-33, 50.5414) construction
  line L13 (-55, 9) -> (-55, 50) construction
  point P0 (-33.54, -25)
  point P1 (-61.54, -25)
  point P2 (55, 16.03)
  point P3 (33, 16.03)
  point P4 (11, 16.03)
  point P5 (-11, 16.03)
  point P6 (-33, 16.03)
  point P7 (-55, 16.03)
  point P8 (-55, 43.97)
  point P9 (-33, 43.97)
  point P10 (-11, 43.97)
  point P11 (11, 43.97)
  point P12 (33, 43.97)
  point P13 (55, 43.97)
  dimension "d150" = 30
  dimension "d151" = 11
  dimension "d152" = 17
  dimension "d153" = 30
  dimension "d154" = 13.97
  dimension "d155" = 13.97
  dimension "d156" = 11
  dimension "d157" = 11
  dimension "d158" = 22
  dimension "d159" = 22
  dimension "d160" = 22
  dimension "d161" = 22
  constraint horizontal L0
  constraint perpendicular L1 L2
  constraint vertical L4
  constraint coincident P0 A0.centre
  constraint coincident L4 P1
  constraint coincident L0 P1
  constraint horizontal L5
  constraint horizontal L6
  constraint horizontal L7
  constraint perpendicular L7 L8
  constraint perpendicular L7 L9
  constraint perpendicular L7 L10
  constraint perpendicular L7 L11
  constraint perpendicular L5 L12
  constraint perpendicular L7 L13
  constraint coincident L6 P2
  constraint coincident L10 P2
  constraint coincident L6 P3
  constraint coincident L9 P3
  constraint coincident L6 P4
  constraint coincident L8 P4
  constraint coincident L6 P5
  constraint coincident L11 P5
  constraint coincident L6 P6
  constraint coincident L12 P6
  constraint coincident L13 P7
  constraint coincident L6 P7
  constraint coincident L13 P8
  constraint coincident L7 P8
  constraint coincident L12 P9
  constraint coincident L7 P9
  constraint coincident L11 P10
  constraint coincident L7 P10
  constraint coincident L7 P11
  constraint coincident L8 P11
  constraint coincident L7 P12
  constraint coincident L9 P12
  constraint coincident L7 P13
  constraint coincident L10 P13
  measures "d150" distance of L0 L1
  measures "d151" distance of L2 L3
  measures "d152" distance of L3 L4
  measures "d153" distance of L5 origin
  measures "d154" distance of L5 L6
  measures "d155" distance of L5 L7
  measures "d156" distance of origin L8
  measures "d157" distance of origin L11
  measures "d158" distance of L11 L12
  measures "d159" distance of L12 L13
  measures "d160" distance of L8 L9
  measures "d161" distance of L9 L10
hole "Bohrung9" at (-55, -43.97, 10.3) at (-33, -43.97, 10.3) at (-11, -43.97, 10.3) at (11, -43.97, 10.3) at (33, -43.97, 10.3) at (55, -43.97, 10.3) at (55, -16.03, 10.3) at (33, -16.03, 10.3) at (11, -16.03, 10.3) at (-11, -16.03, 10.3) at (-33, -16.03, 10.3) at (-55, -16.03, 10.3) at (33.54, 25, 10.3) at (61.54, 25, 10.3) direction (0, 0, -1) diameter 3.5 depth 8.5 tip angle 180 bodies 13 14 15 16 17 18 19 20 21 22 23 24 25 26
ref_plane "Arbeitsebene1" through (0, 0, 6) normal (0, 0, 1) x (1, 0, 0)
sketch "Skizze4" plane through (0, 0, 6) normal (0, 0, 1) x (1, 0, 0)
  line L0 (13.4239, 25) -> (80.4396, 25) construction
  line L1 (61.54, 36.4048) -> (61.54, 10) construction
  line L2 (33.54, 38.5292) -> (33.54, 7.8217) construction
  line L3 (44.54, 45) -> (44.54, 0)
  line L4 (0, 60) -> (0, -58.8077) construction
  line L5 (-91.9293, -30) -> (93.6675, -30) construction
  line L6 (55, -6.4698) -> (55, -54.3658) construction
  line L7 (33, -5.8904) -> (33, -58.6146) construction
  line L8 (11, -5.5042) -> (11, -56.6833) construction
  line L9 (-11, -9.1736) -> (-11, -58.6146) construction
  line L10 (-33, -7.8217) -> (-33, -60) construction
  line L11 (-55, -8.7874) -> (-55, -56.1039) construction
  line L12 (-64.1831, -16.03) -> (77.3903, -16.03) construction
  line L13 (-65.078, -43.97) -> (77.5693, -43.97) construction
  line L14 (63.2432, 22.05) -> (64.9464, 25)
  line L15 (64.9464, 25) -> (63.2432, 27.95)
  line L16 (63.2432, 27.95) -> (59.8368, 27.95)
  line L17 (59.8368, 27.95) -> (58.1336, 25)
  line L18 (58.1336, 25) -> (59.8368, 22.05)
  line L19 (59.8368, 22.05) -> (63.2432, 22.05)
  line L20 (35.2432, 22.05) -> (36.9464, 25)
  line L21 (36.9464, 25) -> (35.2432, 27.95)
  line L22 (35.2432, 27.95) -> (31.8368, 27.95)
  line L23 (31.8368, 27.95) -> (30.1336, 25)
  line L24 (30.1336, 25) -> (31.8368, 22.05)
  line L25 (31.8368, 22.05) -> (35.2432, 22.05)
  line L26 (56.7032, -18.98) -> (58.4064, -16.03)
  line L27 (58.4064, -16.03) -> (56.7032, -13.08)
  line L28 (56.7032, -13.08) -> (53.2968, -13.08)
  line L29 (53.2968, -13.08) -> (51.5936, -16.03)
  line L30 (51.5936, -16.03) -> (53.2968, -18.98)
  line L31 (53.2968, -18.98) -> (56.7032, -18.98)
  line L32 (34.7032, -18.98) -> (36.4064, -16.03)
  line L33 (36.4064, -16.03) -> (34.7032, -13.08)
  line L34 (34.7032, -13.08) -> (31.2968, -13.08)
  line L35 (31.2968, -13.08) -> (29.5936, -16.03)
  line L36 (29.5936, -16.03) -> (31.2968, -18.98)
  line L37 (31.2968, -18.98) -> (34.7032, -18.98)
  line L38 (12.7032, -18.98) -> (14.4064, -16.03)
  line L39 (14.4064, -16.03) -> (12.7032, -13.08)
  line L40 (12.7032, -13.08) -> (9.2968, -13.08)
  line L41 (9.2968, -13.08) -> (7.5936, -16.03)
  line L42 (7.5936, -16.03) -> (9.2968, -18.98)
  line L43 (9.2968, -18.98) -> (12.7032, -18.98)
  line L44 (-9.2968, -18.98) -> (-7.5936, -16.03)
  line L45 (-7.5936, -16.03) -> (-9.2968, -13.08)
  line L46 (-9.2968, -13.08) -> (-12.7032, -13.08)
  line L47 (-12.7032, -13.08) -> (-14.4064, -16.03)
  line L48 (-14.4064, -16.03) -> (-12.7032, -18.98)
  line L49 (-12.7032, -18.98) -> (-9.2968, -18.98)
  line L50 (-31.2968, -18.98) -> (-29.5936, -16.03)
  line L51 (-29.5936, -16.03) -> (-31.2968, -13.08)
  line L52 (-31.2968, -13.08) -> (-34.7032, -13.08)
  line L53 (-34.7032, -13.08) -> (-36.4064, -16.03)
  line L54 (-36.4064, -16.03) -> (-34.7032, -18.98)
  line L55 (-34.7032, -18.98) -> (-31.2968, -18.98)
  line L56 (-53.2968, -18.98) -> (-51.5936, -16.03)
  line L57 (-51.5936, -16.03) -> (-53.2968, -13.08)
  line L58 (-53.2968, -13.08) -> (-56.7032, -13.08)
  line L59 (-56.7032, -13.08) -> (-58.4064, -16.03)
  line L60 (-58.4064, -16.03) -> (-56.7032, -18.98)
  line L61 (-56.7032, -18.98) -> (-53.2968, -18.98)
  line L62 (-53.2968, -46.92) -> (-51.5936, -43.97)
  line L63 (-51.5936, -43.97) -> (-53.2968, -41.02)
  line L64 (-53.2968, -41.02) -> (-56.7032, -41.02)
  line L65 (-56.7032, -41.02) -> (-58.4064, -43.97)
  line L66 (-58.4064, -43.97) -> (-56.7032, -46.92)
  line L67 (-56.7032, -46.92) -> (-53.2968, -46.92)
  line L68 (-31.2968, -46.92) -> (-29.5936, -43.97)
  line L69 (-29.5936, -43.97) -> (-31.2968, -41.02)
  line L70 (-31.2968, -41.02) -> (-34.7032, -41.02)
  line L71 (-34.7032, -41.02) -> (-36.4064, -43.97)
  line L72 (-36.4064, -43.97) -> (-34.7032, -46.92)
  line L73 (-34.7032, -46.92) -> (-31.2968, -46.92)
  line L74 (-9.2968, -46.92) -> (-7.5936, -43.97)
  line L75 (-7.5936, -43.97) -> (-9.2968, -41.02)
  line L76 (-9.2968, -41.02) -> (-12.7032, -41.02)
  line L77 (-12.7032, -41.02) -> (-14.4064, -43.97)
  line L78 (-14.4064, -43.97) -> (-12.7032, -46.92)
  line L79 (-12.7032, -46.92) -> (-9.2968, -46.92)
  line L80 (12.7032, -46.92) -> (14.4064, -43.97)
  line L81 (14.4064, -43.97) -> (12.7032, -41.02)
  line L82 (12.7032, -41.02) -> (9.2968, -41.02)
  line L83 (9.2968, -41.02) -> (7.5936, -43.97)
  line L84 (7.5936, -43.97) -> (9.2968, -46.92)
  line L85 (9.2968, -46.92) -> (12.7032, -46.92)
  line L86 (34.7032, -46.92) -> (36.4064, -43.97)
  line L87 (36.4064, -43.97) -> (34.7032, -41.02)
  line L88 (34.7032, -41.02) -> (31.2968, -41.02)
  line L89 (31.2968, -41.02) -> (29.5936, -43.97)
  line L90 (29.5936, -43.97) -> (31.2968, -46.92)
  line L91 (31.2968, -46.92) -> (34.7032, -46.92)
  line L92 (56.7032, -46.92) -> (58.4064, -43.97)
  line L93 (58.4064, -43.97) -> (56.7032, -41.02)
  line L94 (56.7032, -41.02) -> (53.2968, -41.02)
  line L95 (53.2968, -41.02) -> (51.5936, -43.97)
  line L96 (51.5936, -43.97) -> (53.2968, -46.92)
  line L97 (53.2968, -46.92) -> (56.7032, -46.92)
  point P0 (33.54, 25)
  point P1 (61.54, 25)
  point P2 (55, -16.03)
  point P3 (33, -16.03)
  point P4 (11, -16.03)
  point P5 (-11, -16.03)
  point P6 (-33, -16.03)
  point P7 (-55, -16.03)
  point P8 (-55, -43.97)
  point P9 (-33, -43.97)
  point P10 (-11, -43.97)
  point P11 (11, -43.97)
  point P12 (33, -43.97)
  point P13 (55, -43.97)
  point P14 (61.54, 25)
  point P15 (33.54, 25)
  point P16 (55, -16.03)
  point P17 (33, -16.03)
  point P18 (11, -16.03)
  point P19 (-11, -16.03)
  point P20 (-33, -16.03)
  point P21 (-55, -16.03)
  point P22 (-55, -43.97)
  point P23 (-33, -43.97)
  point P24 (-11, -43.97)
  point P25 (11, -43.97)
  point P26 (33, -43.97)
  point P27 (55, -43.97)
  dimension "d166" = 25
  dimension "d167" = 44.54
  dimension "d168" = 11
  dimension "d169" = 17
  dimension "d170" = 30
  dimension "d171" = 11
  dimension "d173" = 22
  dimension "d174" = 22
  dimension "d175" = 11
  dimension "d176" = 22
  dimension "d177" = 22
  dimension "d178" = 13.97
  dimension "d179" = 13.97
  dimension "d180" = 5.9
  dimension "d181" = 5.9
  dimension "d182" = 5.9
  dimension "d183" = 5.9
  dimension "d184" = 5.9
  dimension "d185" = 5.9
  dimension "d186" = 5.9
  dimension "d187" = 5.9
  dimension "d188" = 5.9
  dimension "d189" = 5.9
  dimension "d190" = 5.9
  dimension "d191" = 5.9
  dimension "d192" = 5.9
  dimension "d193" = 5.9
  constraint horizontal L0
  constraint vertical L1
  constraint vertical L2
  constraint vertical L3
  constraint vertical L4
  constraint coincident L2 P15
  constraint coincident L0 P15
  constraint coincident L1 P14
  constraint coincident L0 P14
  constraint horizontal L5
  constraint perpendicular L0 L6
  constraint vertical L7
  constraint vertical L8
  constraint vertical L9
  constraint vertical L10
  constraint vertical L11
  constraint horizontal L12
  constraint horizontal L13
  constraint coincident L6 P16
  constraint coincident L12 P16
  constraint coincident L12 P17
  constraint coincident L7 P17
  constraint coincident L12 P18
  constraint coincident L8 P18
  constraint coincident L12 P19
  constraint coincident L9 P19
  constraint coincident L12 P20
  constraint coincident L10 P20
  constraint coincident L12 P21
  constraint coincident L11 P21
  constraint coincident L13 P22
  constraint coincident L11 P22
  constraint coincident L10 P23
  constraint coincident L13 P23
  constraint coincident L13 P24
  constraint coincident L9 P24
  constraint coincident L13 P25
  constraint coincident L8 P25
  constraint coincident L13 P26
  constraint coincident L7 P26
  constraint coincident L13 P27
  constraint coincident L6 P27
  constraint coincident P14 P1
  constraint coincident P15 P0
  constraint coincident P16 P2
  constraint coincident P17 P3
  constraint coincident P18 P4
  constraint coincident P19 P5
  constraint coincident P20 P6
  constraint coincident P21 P7
  constraint coincident P22 P8
  constraint coincident P23 P9
  constraint coincident P24 P10
  constraint coincident P25 P11
  constraint coincident P26 P12
  constraint coincident P27 P13
  measures "d166" distance of L0 origin
  measures "d167" distance of L3 L4
  measures "d168" distance of L2 L3
  measures "d169" distance of L1 L3
  measures "d170" distance of L5 origin
  measures "d171" distance of L4 L9
  measures "d173" distance of L9 L10
  measures "d174" distance of L10 L11
  measures "d175" distance of L4 L8
  measures "d176" distance of L7 L8
  measures "d177" distance of L6 L7
  measures "d178" distance of L5 L12
  measures "d179" distance of L5 L13
  measures "d180" distance of L16 L19
  measures "d181" distance of L22 L25
  measures "d182" distance of L28 L31
  measures "d183" distance of L34 L37
  measures "d184" distance of L40 L43
  measures "d185" distance of L46 L49
  measures "d186" distance of L52 L55
  measures "d187" distance of L58 L61
  measures "d188" distance of L64 L67
  measures "d189" distance of L70 L73
  measures "d190" distance of L76 L79
  measures "d191" distance of L82 L85
  measures "d192" distance of L88 L91
  measures "d193" distance of L94 L97
extrude "Extrusion11" cut sketch "Skizze4" along normal blind 2.6 bodies 13 14 15 16 17 18 19 20 21 22 23 24 25 26
ref_plane "Arbeitsebene2" through (0, 0, 6) normal (0, 0, 1) x (1, 0, 0)